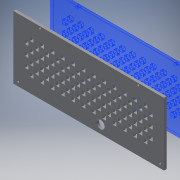
# Autodesk Inventor part: Gehaeuse_IN12_Rueckwand_V1.1
Saved by Autodesk Inventor 2019 (Build 230136000, 136)
## iProperties
Created: 2019-11-09
Part Number: Gehaeuse_IN12_Rueckwand_V1.1
Material: Generisch
Document SubType Name: Modeling
Designer: grubi
Density: 1 g/cm^3
Appearance: Vorgabe
Author: grubi
Autodesk Inventor part; units mm, degrees
ref_plane "YZ Plane" through (0, 0, 0) normal (1, 0, 0) x (0, 1, 0)
ref_plane "XZ Plane" through (0, 0, 0) normal (0, 1, 0) x (-1, 0, 0)
ref_plane "XY Plane" through (0, 0, 0) normal (0, 0, 1) x (1, 0, 0)
sketch "Skizze1" plane through (0, 0, 0) normal (0, 0, 1) x (1, 0, 0)
  line L0 (-87.25, -36.5) -> (87.25, -36.5)
  line L1 (87.25, -36.5) -> (87.25, 36.5)
  line L2 (87.25, 36.5) -> (-87.25, 36.5)
  line L3 (-87.25, 36.5) -> (-87.25, -36.5)
  line L4 (-87.25, -36.5) -> (87.25, 36.5) construction
  line L5 (87.25, -36.5) -> (-87.25, 36.5) construction
  circle A0 centre (-82.267, -31.5) radius 1.45
  line L6 (0, -36.5) -> (0, 36.5) construction
  circle A1 centre (82.267, -31.5) radius 1.45
  circle A2 centre (13.75, -27) radius 4.75
  point P0 (0, 0)
  dimension "d2" = 174.5
  dimension "d3" = 73
  dimension "d4" = 2.9
  dimension "d5" = 5
  dimension "d6" = 164.534
  dimension "d7" = 9.5
  dimension "d8" = 73.5
  dimension "d9" = 9.5
  constraints: 14 end point, 4 midpoint, 3 centre point, 2 parallel, 1 horizontal, 1 perpendicular, 1 symmetric about line, 1 other
  measures "d2" distance of L0.start L0.end
  measures "d3" distance of L0.end L1.end
  measures "d4" diameter of A0
  measures "d5" distance from line of A0.centre L0
  measures "d6" distance of A1.centre A0.centre
  measures "d7" diameter of A2
  measures "d8" distance from line of A2.centre L1
  measures "d9" distance from line of A2.centre L0
extrude "Extrusion1" add sketch "Skizze1" along normal blind 3
sketch "Skizze2" plane through (0, 0, 3) normal (0, 0, 1) x (1, 0, 0)
  line L0 (-2, -2) -> (2, -2)
  line L1 (2, -2) -> (2, 2)
  line L2 (2, 2) -> (-2, 2)
  line L3 (-2, 2) -> (-2, -2)
  line L4 (-2, -2) -> (2, 2) construction
  line L5 (2, -2) -> (-2, 2) construction
  line L6 (-87.25, -36.5) -> (87.25, -36.5) projected
  line L7 (-87.25, 36.5) -> (-87.25, -36.5) projected
  line L8 (-14, -2) -> (-10, -2)
  line L9 (-10, -2) -> (-10, 2)
  line L10 (-10, 2) -> (-14, 2)
  line L11 (-14, 2) -> (-14, -2)
  line L12 (-14, -2) -> (-10, 2) construction
  line L13 (-10, -2) -> (-14, 2) construction
  line L14 (-26, -2) -> (-22, -2)
  line L15 (-22, -2) -> (-22, 2)
  line L16 (-22, 2) -> (-26, 2)
  line L17 (-26, 2) -> (-26, -2)
  line L18 (-26, -2) -> (-22, 2) construction
  line L19 (-22, -2) -> (-26, 2) construction
  line L20 (-38, -2) -> (-34, -2)
  line L21 (-34, -2) -> (-34, 2)
  line L22 (-34, 2) -> (-38, 2)
  line L23 (-38, 2) -> (-38, -2)
  line L24 (-38, -2) -> (-34, 2) construction
  line L25 (-34, -2) -> (-38, 2) construction
  line L26 (-50, -2) -> (-46, -2)
  line L27 (-46, -2) -> (-46, 2)
  line L28 (-46, 2) -> (-50, 2)
  line L29 (-50, 2) -> (-50, -2)
  line L30 (-50, -2) -> (-46, 2) construction
  line L31 (-46, -2) -> (-50, 2) construction
  line L32 (-62, -2) -> (-58, -2)
  line L33 (-58, -2) -> (-58, 2)
  line L34 (-58, 2) -> (-62, 2)
  line L35 (-62, 2) -> (-62, -2)
  line L36 (-62, -2) -> (-58, 2) construction
  line L37 (-58, -2) -> (-62, 2) construction
  line L38 (-74, -2) -> (-70, -2)
  line L39 (-70, -2) -> (-70, 2)
  line L40 (-70, 2) -> (-74, 2)
  line L41 (-74, 2) -> (-74, -2)
  line L42 (-74, -2) -> (-70, 2) construction
  line L43 (-70, -2) -> (-74, 2) construction
  line L44 (-2, -14) -> (2, -14)
  line L45 (2, -14) -> (2, -10)
  line L46 (2, -10) -> (-2, -10)
  line L47 (-2, -10) -> (-2, -14)
  line L48 (-2, -14) -> (2, -10) construction
  line L49 (2, -14) -> (-2, -10) construction
  line L50 (-14, -14) -> (-10, -14)
  line L51 (-10, -14) -> (-10, -10)
  line L52 (-10, -10) -> (-14, -10)
  line L53 (-14, -10) -> (-14, -14)
  line L54 (-14, -14) -> (-10, -10) construction
  line L55 (-10, -14) -> (-14, -10) construction
  line L56 (-26, -14) -> (-22, -14)
  line L57 (-22, -14) -> (-22, -10)
  line L58 (-22, -10) -> (-26, -10)
  line L59 (-26, -10) -> (-26, -14)
  line L60 (-26, -14) -> (-22, -10) construction
  line L61 (-22, -14) -> (-26, -10) construction
  line L62 (-38, -14) -> (-34, -14)
  line L63 (-34, -14) -> (-34, -10)
  line L64 (-34, -10) -> (-38, -10)
  line L65 (-38, -10) -> (-38, -14)
  line L66 (-38, -14) -> (-34, -10) construction
  line L67 (-34, -14) -> (-38, -10) construction
  line L68 (-50, -14) -> (-46, -14)
  line L69 (-46, -14) -> (-46, -10)
  line L70 (-46, -10) -> (-50, -10)
  line L71 (-50, -10) -> (-50, -14)
  line L72 (-50, -14) -> (-46, -10) construction
  line L73 (-46, -14) -> (-50, -10) construction
  line L74 (-62, -14) -> (-58, -14)
  line L75 (-58, -14) -> (-58, -10)
  line L76 (-58, -10) -> (-62, -10)
  line L77 (-62, -10) -> (-62, -14)
  line L78 (-62, -14) -> (-58, -10) construction
  line L79 (-58, -14) -> (-62, -10) construction
  line L80 (-74, -14) -> (-70, -14)
  line L81 (-70, -14) -> (-70, -10)
  line L82 (-70, -10) -> (-74, -10)
  line L83 (-74, -10) -> (-74, -14)
  line L84 (-74, -14) -> (-70, -10) construction
  line L85 (-70, -14) -> (-74, -10) construction
  line L86 (-8, -8) -> (-4, -8)
  line L87 (-4, -8) -> (-4, -4)
  line L88 (-4, -4) -> (-8, -4)
  line L89 (-8, -4) -> (-8, -8)
  line L90 (-8, -8) -> (-4, -4) construction
  line L91 (-4, -8) -> (-8, -4) construction
  line L92 (-16, -4) -> (-20, -4)
  line L93 (-20, -8) -> (-16, -4) construction
  line L94 (-20, -8) -> (-16, -8)
  line L95 (-16, -8) -> (-20, -4) construction
  line L96 (-16, -8) -> (-16, -4)
  line L97 (-20, -4) -> (-20, -8)
  line L98 (-28, -4) -> (-32, -4)
  line L99 (-32, -8) -> (-28, -4) construction
  line L100 (-32, -8) -> (-28, -8)
  line L101 (-28, -8) -> (-32, -4) construction
  line L102 (-28, -8) -> (-28, -4)
  line L103 (-32, -4) -> (-32, -8)
  line L104 (-40, -4) -> (-44, -4)
  line L105 (-44, -8) -> (-40, -4) construction
  line L106 (-44, -8) -> (-40, -8)
  line L107 (-40, -8) -> (-44, -4) construction
  line L108 (-40, -8) -> (-40, -4)
  line L109 (-44, -4) -> (-44, -8)
  line L110 (-52, -4) -> (-56, -4)
  line L111 (-56, -8) -> (-52, -4) construction
  line L112 (-56, -8) -> (-52, -8)
  line L113 (-52, -8) -> (-56, -4) construction
  line L114 (-52, -8) -> (-52, -4)
  line L115 (-56, -4) -> (-56, -8)
  line L116 (-64, -4) -> (-68, -4)
  line L117 (-68, -8) -> (-64, -4) construction
  line L118 (-68, -8) -> (-64, -8)
  line L119 (-64, -8) -> (-68, -4) construction
  line L120 (-64, -8) -> (-64, -4)
  line L121 (-68, -4) -> (-68, -8)
  line L122 (-4, -16) -> (-8, -16)
  line L123 (-8, -20) -> (-4, -16) construction
  line L124 (-8, -20) -> (-4, -20)
  line L125 (-4, -20) -> (-8, -16) construction
  line L126 (-4, -20) -> (-4, -16)
  line L127 (-8, -16) -> (-8, -20)
  line L128 (-16, -16) -> (-20, -16)
  line L129 (-20, -20) -> (-16, -16) construction
  line L130 (-20, -20) -> (-16, -20)
  line L131 (-16, -20) -> (-20, -16) construction
  line L132 (-16, -20) -> (-16, -16)
  line L133 (-20, -16) -> (-20, -20)
  line L134 (-28, -16) -> (-32, -16)
  line L135 (-32, -20) -> (-28, -16) construction
  line L136 (-32, -20) -> (-28, -20)
  line L137 (-28, -20) -> (-32, -16) construction
  line L138 (-28, -20) -> (-28, -16)
  line L139 (-32, -16) -> (-32, -20)
  line L140 (-40, -16) -> (-44, -16)
  line L141 (-44, -20) -> (-40, -16) construction
  line L142 (-44, -20) -> (-40, -20)
  line L143 (-40, -20) -> (-44, -16) construction
  line L144 (-40, -20) -> (-40, -16)
  line L145 (-44, -16) -> (-44, -20)
  line L146 (-52, -16) -> (-56, -16)
  line L147 (-56, -20) -> (-52, -16) construction
  line L148 (-56, -20) -> (-52, -20)
  line L149 (-52, -20) -> (-56, -16) construction
  line L150 (-52, -20) -> (-52, -16)
  line L151 (-56, -16) -> (-56, -20)
  line L152 (-64, -16) -> (-68, -16)
  line L153 (-68, -20) -> (-64, -16) construction
  line L154 (-68, -20) -> (-64, -20)
  line L155 (-64, -20) -> (-68, -16) construction
  line L156 (-64, -20) -> (-64, -16)
  line L157 (-68, -16) -> (-68, -20)
  line L158 (0, -36.5) -> (0, 36.5) construction
  line L159 (87.25, 36.5) -> (-87.25, 36.5) projected
  line L160 (2, -2) -> (-2, -2)
  line L161 (-2, -2) -> (-2, 2)
  line L162 (-2, 2) -> (2, 2)
  line L163 (2, 2) -> (2, -2)
  line L164 (2, -2) -> (-2, 2) construction
  line L165 (-2, -2) -> (2, 2) construction
  line L166 (14, -2) -> (10, -2)
  line L167 (10, -2) -> (10, 2)
  line L168 (10, 2) -> (14, 2)
  line L169 (14, 2) -> (14, -2)
  line L170 (14, -2) -> (10, 2) construction
  line L171 (10, -2) -> (14, 2) construction
  line L172 (26, -2) -> (22, -2)
  line L173 (22, -2) -> (22, 2)
  line L174 (22, 2) -> (26, 2)
  line L175 (26, 2) -> (26, -2)
  line L176 (26, -2) -> (22, 2) construction
  line L177 (22, -2) -> (26, 2) construction
  line L178 (38, -2) -> (34, -2)
  line L179 (34, -2) -> (34, 2)
  line L180 (34, 2) -> (38, 2)
  line L181 (38, 2) -> (38, -2)
  line L182 (38, -2) -> (34, 2) construction
  line L183 (34, -2) -> (38, 2) construction
  line L184 (50, -2) -> (46, -2)
  line L185 (46, -2) -> (46, 2)
  line L186 (46, 2) -> (50, 2)
  line L187 (50, 2) -> (50, -2)
  line L188 (50, -2) -> (46, 2) construction
  line L189 (46, -2) -> (50, 2) construction
  line L190 (62, -2) -> (58, -2)
  line L191 (58, -2) -> (58, 2)
  line L192 (58, 2) -> (62, 2)
  line L193 (62, 2) -> (62, -2)
  line L194 (62, -2) -> (58, 2) construction
  line L195 (58, -2) -> (62, 2) construction
  line L196 (74, -2) -> (70, -2)
  line L197 (70, -2) -> (70, 2)
  line L198 (70, 2) -> (74, 2)
  line L199 (74, 2) -> (74, -2)
  line L200 (74, -2) -> (70, 2) construction
  line L201 (70, -2) -> (74, 2) construction
  line L202 (2, -14) -> (-2, -14)
  line L203 (-2, -14) -> (-2, -10)
  line L204 (-2, -10) -> (2, -10)
  line L205 (2, -10) -> (2, -14)
  line L206 (2, -14) -> (-2, -10) construction
  line L207 (-2, -14) -> (2, -10) construction
  line L208 (14, -14) -> (10, -14)
  line L209 (10, -14) -> (10, -10)
  line L210 (10, -10) -> (14, -10)
  line L211 (14, -10) -> (14, -14)
  line L212 (14, -14) -> (10, -10) construction
  line L213 (10, -14) -> (14, -10) construction
  line L214 (26, -14) -> (22, -14)
  line L215 (22, -14) -> (22, -10)
  line L216 (22, -10) -> (26, -10)
  line L217 (26, -10) -> (26, -14)
  line L218 (26, -14) -> (22, -10) construction
  line L219 (22, -14) -> (26, -10) construction
  line L220 (38, -14) -> (34, -14)
  line L221 (34, -14) -> (34, -10)
  line L222 (34, -10) -> (38, -10)
  line L223 (38, -10) -> (38, -14)
  line L224 (38, -14) -> (34, -10) construction
  line L225 (34, -14) -> (38, -10) construction
  line L226 (50, -14) -> (46, -14)
  line L227 (46, -14) -> (46, -10)
  line L228 (46, -10) -> (50, -10)
  line L229 (50, -10) -> (50, -14)
  line L230 (50, -14) -> (46, -10) construction
  line L231 (46, -14) -> (50, -10) construction
  line L232 (62, -14) -> (58, -14)
  line L233 (58, -14) -> (58, -10)
  line L234 (58, -10) -> (62, -10)
  line L235 (62, -10) -> (62, -14)
  line L236 (62, -14) -> (58, -10) construction
  line L237 (58, -14) -> (62, -10) construction
  line L238 (74, -14) -> (70, -14)
  line L239 (70, -14) -> (70, -10)
  line L240 (70, -10) -> (74, -10)
  line L241 (74, -10) -> (74, -14)
  line L242 (74, -14) -> (70, -10) construction
  line L243 (70, -14) -> (74, -10) construction
  line L244 (8, -8) -> (4, -8)
  line L245 (4, -8) -> (4, -4)
  line L246 (4, -4) -> (8, -4)
  line L247 (8, -8) -> (4, -4) construction
  line L248 (4, -8) -> (8, -4) construction
  line L249 (8, -4) -> (8, -8)
  line L250 (16, -4) -> (20, -4)
  line L251 (20, -8) -> (16, -4) construction
  line L252 (20, -8) -> (16, -8)
  line L253 (16, -8) -> (20, -4) construction
  line L254 (16, -8) -> (16, -4)
  line L255 (20, -4) -> (20, -8)
  line L256 (28, -4) -> (32, -4)
  line L257 (32, -8) -> (28, -4) construction
  line L258 (32, -8) -> (28, -8)
  line L259 (28, -8) -> (32, -4) construction
  line L260 (28, -8) -> (28, -4)
  line L261 (32, -4) -> (32, -8)
  line L262 (40, -4) -> (44, -4)
  line L263 (44, -8) -> (40, -4) construction
  line L264 (44, -8) -> (40, -8)
  line L265 (40, -8) -> (44, -4) construction
  line L266 (40, -8) -> (40, -4)
  line L267 (44, -4) -> (44, -8)
  line L268 (52, -4) -> (56, -4)
  line L269 (56, -8) -> (52, -4) construction
  line L270 (56, -8) -> (52, -8)
  line L271 (52, -8) -> (56, -4) construction
  line L272 (52, -8) -> (52, -4)
  line L273 (56, -4) -> (56, -8)
  line L274 (64, -4) -> (68, -4)
  line L275 (68, -8) -> (64, -4) construction
  line L276 (68, -8) -> (64, -8)
  line L277 (64, -8) -> (68, -4) construction
  line L278 (64, -8) -> (64, -4)
  line L279 (68, -4) -> (68, -8)
  line L280 (4, -16) -> (8, -16)
  line L281 (8, -20) -> (4, -16) construction
  line L282 (8, -20) -> (4, -20)
  line L283 (4, -20) -> (8, -16) construction
  line L284 (4, -20) -> (4, -16)
  line L285 (8, -16) -> (8, -20)
  line L286 (16, -16) -> (20, -16)
  line L287 (20, -20) -> (16, -16) construction
  line L288 (20, -20) -> (16, -20)
  line L289 (16, -20) -> (20, -16) construction
  line L290 (16, -20) -> (16, -16)
  line L291 (20, -16) -> (20, -20)
  line L292 (28, -16) -> (32, -16)
  line L293 (32, -20) -> (28, -16) construction
  line L294 (32, -20) -> (28, -20)
  line L295 (28, -20) -> (32, -16) construction
  line L296 (28, -20) -> (28, -16)
  line L297 (32, -16) -> (32, -20)
  line L298 (40, -16) -> (44, -16)
  line L299 (44, -20) -> (40, -16) construction
  line L300 (44, -20) -> (40, -20)
  line L301 (40, -20) -> (44, -16) construction
  line L302 (40, -20) -> (40, -16)
  line L303 (44, -16) -> (44, -20)
  line L304 (52, -16) -> (56, -16)
  line L305 (56, -20) -> (52, -16) construction
  line L306 (56, -20) -> (52, -20)
  line L307 (52, -20) -> (56, -16) construction
  line L308 (52, -20) -> (52, -16)
  line L309 (56, -16) -> (56, -20)
  line L310 (64, -16) -> (68, -16)
  line L311 (68, -20) -> (64, -16) construction
  line L312 (68, -20) -> (64, -20)
  line L313 (64, -20) -> (68, -16) construction
  line L314 (64, -20) -> (64, -16)
  line L315 (68, -16) -> (68, -20)
  line L316 (-87.25, 0) -> (87.25, 0) construction
  line L317 (-2, 2) -> (2, 2)
  line L318 (2, 2) -> (2, -2)
  line L319 (2, -2) -> (-2, -2)
  line L320 (-2, -2) -> (-2, 2)
  line L321 (-2, 2) -> (2, -2) construction
  line L322 (2, 2) -> (-2, -2) construction
  line L323 (-14, 2) -> (-10, 2)
  line L324 (-10, 2) -> (-10, -2)
  line L325 (-10, -2) -> (-14, -2)
  line L326 (-14, -2) -> (-14, 2)
  line L327 (-14, 2) -> (-10, -2) construction
  line L328 (-10, 2) -> (-14, -2) construction
  line L329 (-26, 2) -> (-22, 2)
  line L330 (-22, 2) -> (-22, -2)
  line L331 (-22, -2) -> (-26, -2)
  line L332 (-26, -2) -> (-26, 2)
  line L333 (-26, 2) -> (-22, -2) construction
  line L334 (-22, 2) -> (-26, -2) construction
  line L335 (-38, 2) -> (-34, 2)
  line L336 (-34, 2) -> (-34, -2)
  line L337 (-34, -2) -> (-38, -2)
  line L338 (-38, -2) -> (-38, 2)
  line L339 (-38, 2) -> (-34, -2) construction
  line L340 (-34, 2) -> (-38, -2) construction
  line L341 (-50, 2) -> (-46, 2)
  line L342 (-46, 2) -> (-46, -2)
  line L343 (-46, -2) -> (-50, -2)
  line L344 (-50, -2) -> (-50, 2)
  line L345 (-50, 2) -> (-46, -2) construction
  line L346 (-46, 2) -> (-50, -2) construction
  line L347 (-62, 2) -> (-58, 2)
  line L348 (-58, 2) -> (-58, -2)
  line L349 (-58, -2) -> (-62, -2)
  line L350 (-62, -2) -> (-62, 2)
  line L351 (-62, 2) -> (-58, -2) construction
  line L352 (-58, 2) -> (-62, -2) construction
  line L353 (-74, 2) -> (-70, 2)
  line L354 (-70, 2) -> (-70, -2)
  line L355 (-70, -2) -> (-74, -2)
  line L356 (-74, -2) -> (-74, 2)
  line L357 (-74, 2) -> (-70, -2) construction
  line L358 (-70, 2) -> (-74, -2) construction
  line L359 (-2, 14) -> (2, 14)
  line L360 (2, 14) -> (2, 10)
  line L361 (2, 10) -> (-2, 10)
  line L362 (-2, 10) -> (-2, 14)
  line L363 (-2, 14) -> (2, 10) construction
  line L364 (2, 14) -> (-2, 10) construction
  line L365 (-14, 14) -> (-10, 14)
  line L366 (-10, 14) -> (-10, 10)
  line L367 (-10, 10) -> (-14, 10)
  line L368 (-14, 10) -> (-14, 14)
  line L369 (-14, 14) -> (-10, 10) construction
  line L370 (-10, 14) -> (-14, 10) construction
  line L371 (-26, 14) -> (-22, 14)
  line L372 (-22, 14) -> (-22, 10)
  line L373 (-22, 10) -> (-26, 10)
  line L374 (-26, 10) -> (-26, 14)
  line L375 (-26, 14) -> (-22, 10) construction
  line L376 (-22, 14) -> (-26, 10) construction
  line L377 (-38, 14) -> (-34, 14)
  line L378 (-34, 14) -> (-34, 10)
  line L379 (-34, 10) -> (-38, 10)
  line L380 (-38, 10) -> (-38, 14)
  line L381 (-38, 14) -> (-34, 10) construction
  line L382 (-34, 14) -> (-38, 10) construction
  line L383 (-50, 14) -> (-46, 14)
  line L384 (-46, 14) -> (-46, 10)
  line L385 (-46, 10) -> (-50, 10)
  line L386 (-50, 10) -> (-50, 14)
  line L387 (-50, 14) -> (-46, 10) construction
  line L388 (-46, 14) -> (-50, 10) construction
  line L389 (-62, 14) -> (-58, 14)
  line L390 (-58, 14) -> (-58, 10)
  line L391 (-58, 10) -> (-62, 10)
  line L392 (-62, 10) -> (-62, 14)
  line L393 (-62, 14) -> (-58, 10) construction
  line L394 (-58, 14) -> (-62, 10) construction
  line L395 (-74, 14) -> (-70, 14)
  line L396 (-70, 14) -> (-70, 10)
  line L397 (-70, 10) -> (-74, 10)
  line L398 (-74, 10) -> (-74, 14)
  line L399 (-74, 14) -> (-70, 10) construction
  line L400 (-70, 14) -> (-74, 10) construction
  line L401 (-8, 8) -> (-4, 8)
  line L402 (-4, 8) -> (-4, 4)
  line L403 (-4, 4) -> (-8, 4)
  line L404 (-8, 8) -> (-4, 4) construction
  line L405 (-4, 8) -> (-8, 4) construction
  line L406 (-8, 4) -> (-8, 8)
  line L407 (-16, 4) -> (-20, 4)
  line L408 (-20, 8) -> (-16, 4) construction
  line L409 (-20, 8) -> (-16, 8)
  line L410 (-16, 8) -> (-20, 4) construction
  line L411 (-16, 8) -> (-16, 4)
  line L412 (-20, 4) -> (-20, 8)
  line L413 (-28, 4) -> (-32, 4)
  line L414 (-32, 8) -> (-28, 4) construction
  line L415 (-32, 8) -> (-28, 8)
  line L416 (-28, 8) -> (-32, 4) construction
  line L417 (-28, 8) -> (-28, 4)
  line L418 (-32, 4) -> (-32, 8)
  line L419 (-40, 4) -> (-44, 4)
  line L420 (-44, 8) -> (-40, 4) construction
  line L421 (-44, 8) -> (-40, 8)
  line L422 (-40, 8) -> (-44, 4) construction
  line L423 (-40, 8) -> (-40, 4)
  line L424 (-44, 4) -> (-44, 8)
  line L425 (-52, 4) -> (-56, 4)
  line L426 (-56, 8) -> (-52, 4) construction
  line L427 (-56, 8) -> (-52, 8)
  line L428 (-52, 8) -> (-56, 4) construction
  line L429 (-52, 8) -> (-52, 4)
  line L430 (-56, 4) -> (-56, 8)
  line L431 (-64, 4) -> (-68, 4)
  line L432 (-68, 8) -> (-64, 4) construction
  line L433 (-68, 8) -> (-64, 8)
  line L434 (-64, 8) -> (-68, 4) construction
  line L435 (-64, 8) -> (-64, 4)
  line L436 (-68, 4) -> (-68, 8)
  line L437 (-4, 16) -> (-8, 16)
  line L438 (-8, 20) -> (-4, 16) construction
  line L439 (-8, 20) -> (-4, 20)
  line L440 (-4, 20) -> (-8, 16) construction
  line L441 (-4, 20) -> (-4, 16)
  line L442 (-8, 16) -> (-8, 20)
  line L443 (-16, 16) -> (-20, 16)
  line L444 (-20, 20) -> (-16, 16) construction
  line L445 (-20, 20) -> (-16, 20)
  line L446 (-16, 20) -> (-20, 16) construction
  line L447 (-16, 20) -> (-16, 16)
  line L448 (-20, 16) -> (-20, 20)
  line L449 (-28, 16) -> (-32, 16)
  line L450 (-32, 20) -> (-28, 16) construction
  line L451 (-32, 20) -> (-28, 20)
  line L452 (-28, 20) -> (-32, 16) construction
  line L453 (-28, 20) -> (-28, 16)
  line L454 (-32, 16) -> (-32, 20)
  line L455 (-40, 16) -> (-44, 16)
  line L456 (-44, 20) -> (-40, 16) construction
  line L457 (-44, 20) -> (-40, 20)
  line L458 (-40, 20) -> (-44, 16) construction
  line L459 (-40, 20) -> (-40, 16)
  line L460 (-44, 16) -> (-44, 20)
  line L461 (-52, 16) -> (-56, 16)
  line L462 (-56, 20) -> (-52, 16) construction
  line L463 (-56, 20) -> (-52, 20)
  line L464 (-52, 20) -> (-56, 16) construction
  line L465 (-52, 20) -> (-52, 16)
  line L466 (-56, 16) -> (-56, 20)
  line L467 (-64, 16) -> (-68, 16)
  line L468 (-68, 20) -> (-64, 16) construction
  line L469 (-68, 20) -> (-64, 20)
  line L470 (-64, 20) -> (-68, 16) construction
  line L471 (-64, 20) -> (-64, 16)
  line L472 (-68, 16) -> (-68, 20)
  line L473 (2, 2) -> (-2, 2)
  line L474 (8, 8) -> (4, 8)
  line L475 (4, 8) -> (4, 4)
  line L476 (4, 8) -> (8, 4) construction
  line L477 (8, 8) -> (4, 4) construction
  line L478 (4, 4) -> (8, 4)
  line L479 (-2, 2) -> (-2, -2)
  line L480 (-2, -2) -> (2, -2)
  line L481 (2, -2) -> (2, 2)
  line L482 (2, 2) -> (-2, -2) construction
  line L483 (-2, 2) -> (2, -2) construction
  line L484 (14, 2) -> (10, 2)
  line L485 (10, 2) -> (10, -2)
  line L486 (10, -2) -> (14, -2)
  line L487 (14, -2) -> (14, 2)
  line L488 (10, 2) -> (14, -2) construction
  line L489 (14, 2) -> (10, -2) construction
  line L490 (26, 2) -> (22, 2)
  line L491 (22, 2) -> (22, -2)
  line L492 (22, -2) -> (26, -2)
  line L493 (26, -2) -> (26, 2)
  line L494 (26, 2) -> (22, -2) construction
  line L495 (22, 2) -> (26, -2) construction
  line L496 (38, 2) -> (34, 2)
  line L497 (34, 2) -> (34, -2)
  line L498 (34, -2) -> (38, -2)
  line L499 (32, 8) -> (28, 8)
  line L500 (32, 4) -> (32, 8)
  line L501 (32, 8) -> (28, 4) construction
  line L502 (28, 8) -> (28, 4)
  line L503 (28, 8) -> (32, 4) construction
  line L504 (28, 4) -> (32, 4)
  line L505 (38, -2) -> (38, 2)
  line L506 (38, 2) -> (34, -2) construction
  line L507 (34, 2) -> (38, -2) construction
  line L508 (50, 2) -> (46, 2)
  line L509 (46, 2) -> (46, -2)
  line L510 (46, -2) -> (50, -2)
  line L511 (50, -2) -> (50, 2)
  line L512 (46, 2) -> (50, -2) construction
  line L513 (50, 2) -> (46, -2) construction
  line L514 (8, 16) -> (8, 20)
  line L515 (14, 14) -> (10, 14)
  line L516 (14, 10) -> (14, 14)
  line L517 (10, 14) -> (14, 10) construction
  line L518 (10, 14) -> (10, 10)
  line L519 (14, 14) -> (10, 10) construction
  line L520 (20, 8) -> (16, 8)
  line L521 (16, 4) -> (20, 4)
  line L522 (16, 8) -> (20, 4) construction
  line L523 (20, 4) -> (20, 8)
  line L524 (20, 8) -> (16, 4) construction
  line L525 (10, 10) -> (14, 10)
  line L526 (16, 8) -> (16, 4)
  line L527 (8, 4) -> (8, 8)
  line L528 (26, 14) -> (22, 14)
  line L529 (22, 14) -> (22, 10)
  line L530 (22, 10) -> (26, 10)
  line L531 (26, 14) -> (22, 10) construction
  line L532 (22, 14) -> (26, 10) construction
  line L533 (26, 10) -> (26, 14)
  line L534 (-2, 10) -> (2, 10)
  line L535 (2, 10) -> (2, 14)
  line L536 (2, 14) -> (-2, 10) construction
  line L537 (2, 14) -> (-2, 14)
  line L538 (-2, 14) -> (-2, 10)
  line L539 (-2, 14) -> (2, 10) construction
  line L540 (4, 16) -> (8, 16)
  line L541 (4, 20) -> (8, 16) construction
  line L542 (8, 20) -> (4, 16) construction
  line L543 (8, 20) -> (4, 20)
  line L544 (4, 20) -> (4, 16)
  line L545 (40, 4) -> (44, 4)
  line L546 (44, 4) -> (44, 8)
  line L547 (46, 10) -> (50, 10)
  line L548 (40, 8) -> (40, 4)
  line L549 (44, 8) -> (40, 4) construction
  line L550 (44, 8) -> (40, 8)
  line L551 (50, 14) -> (46, 14)
  line L552 (50, 10) -> (50, 14)
  line L553 (50, 14) -> (46, 10) construction
  line L554 (46, 14) -> (50, 10) construction
  line L555 (46, 14) -> (46, 10)
  line L556 (40, 16) -> (44, 16)
  line L557 (44, 16) -> (44, 20)
  line L558 (40, 20) -> (40, 16)
  line L559 (40, 20) -> (44, 16) construction
  line L560 (44, 20) -> (40, 20)
  line L561 (44, 20) -> (40, 16) construction
  line L562 (40, 8) -> (44, 4) construction
  line L563 (34, 10) -> (38, 10)
  line L564 (38, 14) -> (34, 14)
  line L565 (38, 10) -> (38, 14)
  line L566 (38, 14) -> (34, 10) construction
  line L567 (34, 14) -> (38, 10) construction
  line L568 (34, 14) -> (34, 10)
  line L569 (28, 16) -> (32, 16)
  line L570 (32, 16) -> (32, 20)
  line L571 (28, 20) -> (28, 16)
  line L572 (28, 20) -> (32, 16) construction
  line L573 (32, 20) -> (28, 20)
  line L574 (32, 20) -> (28, 16) construction
  line L575 (16, 16) -> (20, 16)
  line L576 (16, 20) -> (20, 16) construction
  line L577 (20, 16) -> (20, 20)
  line L578 (20, 20) -> (16, 16) construction
  line L579 (20, 20) -> (16, 20)
  line L580 (16, 20) -> (16, 16)
  line L581 (52, 20) -> (52, 16)
  line L582 (52, 16) -> (56, 16)
  line L583 (52, 20) -> (56, 16) construction
  line L584 (56, 20) -> (52, 20)
  line L585 (64, 20) -> (68, 16) construction
  line L586 (68, 20) -> (64, 16) construction
  line L587 (68, 16) -> (68, 20)
  line L588 (56, 20) -> (52, 16) construction
  line L589 (62, 14) -> (58, 14)
  line L590 (58, 14) -> (58, 10)
  line L591 (58, 10) -> (62, 10)
  line L592 (62, 10) -> (62, 14)
  line L593 (62, 14) -> (58, 10) construction
  line L594 (58, 14) -> (62, 10) construction
  line L595 (52, 4) -> (56, 4)
  line L596 (56, 8) -> (52, 4) construction
  line L597 (56, 8) -> (52, 8)
  line L598 (52, 8) -> (56, 4) construction
  line L599 (52, 8) -> (52, 4)
  line L600 (56, 4) -> (56, 8)
  line L601 (64, 4) -> (68, 4)
  line L602 (68, 8) -> (64, 4) construction
  line L603 (68, 8) -> (64, 8)
  line L604 (64, 8) -> (68, 4) construction
  line L605 (64, 8) -> (64, 4)
  line L606 (68, 4) -> (68, 8)
  line L607 (64, 16) -> (68, 16)
  line L608 (56, 16) -> (56, 20)
  line L609 (68, 20) -> (64, 20)
  line L610 (62, 2) -> (58, 2)
  line L611 (58, 2) -> (58, -2)
  line L612 (58, -2) -> (62, -2)
  line L613 (62, -2) -> (62, 2)
  line L614 (62, 2) -> (58, -2) construction
  line L615 (58, 2) -> (62, -2) construction
  line L616 (74, 2) -> (70, 2)
  line L617 (70, 2) -> (70, -2)
  line L618 (70, -2) -> (74, -2)
  line L619 (74, -2) -> (74, 2)
  line L620 (74, 2) -> (70, -2) construction
  line L621 (70, 2) -> (74, -2) construction
  line L622 (74, 14) -> (70, 14)
  line L623 (70, 14) -> (70, 10)
  line L624 (70, 10) -> (74, 10)
  line L625 (74, 10) -> (74, 14)
  line L626 (74, 14) -> (70, 10) construction
  line L627 (70, 14) -> (74, 10) construction
  line L628 (64, 20) -> (64, 16)
  point P0 (0, 0)
  dimension "d12" = 4
  dimension "d13" = 4
  dimension "d16" = 12
  dimension "d19" = 12
  dimension "d26" = 4
  dimension "d27" = 4
  dimension "d28" = 2
  dimension "d29" = 2
  dimension "d32" = 12
  dimension "d35" = 12
  constraints: 1252 end point, 312 symmetric about line, 11 midpoint, 5 horizontal, 4 parallel, 2 perpendicular, 2 vertical, 240 other
  measures "d12" distance of L2.end L0.start
  measures "d13" distance of L0.start L0.end
  measures "d16" distance of L0.start L8.start
  measures "d19" distance of L0.start L44.start
  measures "d26" distance of L88.end L86.start
  measures "d27" distance of L86.start L86.end
  measures "d28" distance between parallel lines of L3 L87
  measures "d29" distance between parallel lines of L88 L0
  measures "d32" distance of L87.end L92.start
  measures "d35" distance of L87.end L122.start
extrude "Extrusion2" cut sketch "Skizze2" against normal through all
sketch "Skizze6" plane through (0, 0, 0) normal (0, 0, -1) x (-1, 0, 0)
  circle A0 centre (-57, 34.5814) radius 1.45 projected
  circle A1 centre (57, 34.5814) radius 1.45 projected
  point P0 (0, 0)
extrude "Extrusion3" cut sketch "Skizze6" against normal up to surface (3 mm away)
